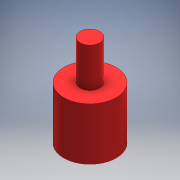
# Autodesk Inventor part: 防振ゴム雄ねじ雌ねじスペーサー
Saved by Autodesk Inventor 2016 (Build 200138000, 138)
## iProperties
Created: 2019-11-20
Part Number: 防振ゴム雄ねじ雌ねじスペーサー
Material: 一般
Document SubType Name: Modeling
Designer: mozar
Mass: 1 g
Surface Area: 3.82521 cm^2
Volume: 0.42858 cm^3
Density: 2.33329 g/cm^3
Appearance: 淡い赤
Author: mozar
Autodesk Inventor part; units mm, degrees
ref_plane "YZ Plane" through (0, 0, 0) normal (1, 0, 0) x (0, 1, 0)
ref_plane "XZ Plane" through (0, 0, 0) normal (0, 1, 0) x (-1, 0, 0)
ref_plane "XY Plane" through (0, 0, 0) normal (0, 0, 1) x (1, 0, 0)
sketch "スケッチ1" plane through (0, 0, 0) normal (0, 0, 1) x (1, 0, 0)
  circle A0 centre (0, 0) radius 4
  circle A1 centre (0, 0) radius 1.5
  dimension "d0" = 8
  dimension "d1" = 3
  constraints: 2 centre point, 2 coincident
  measures "d0" diameter of A0
  measures "d1" diameter of A1
extrude "押し出し1" add sketch "スケッチ1" along normal blind 6 contours A1
extrude "押し出し2" add sketch "スケッチ1" against normal blind 8 contours A0 | A1
sketch "スケッチ2" plane through (0, 0, -8) normal (0, 0, -1) x (-1, 0, 0)
  circle A0 centre (0, 0) radius 4 projected
hole "穴1" at (0, 0, -8) direction (0, 0, 1) diameter 2.5 depth 3 tip angle 118
